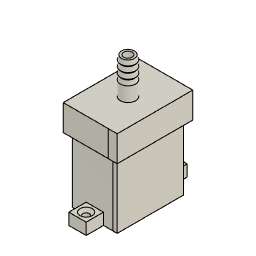
BMP280box v1 (Autodesk Fusion 360 design; units mm, degrees)
Autodesk Fusion 360 part; units mm, degrees
sketch "Sketch1" plane through (0, 0, 0) normal (0, 0, 1) x (1, 0, 0)
  line L0 (0, 0) -> (25, 0)
  line L1 (25, 0) -> (25, 40)
  line L2 (25, 40) -> (0, 40)
  line L3 (0, 40) -> (0, 0)
  line L4 (-3, 43) -> (-3, -3)
  line L5 (-3, -3) -> (28, -3)
  line L6 (28, -3) -> (28, 43)
  line L7 (28, 43) -> (-3, 43)
  line L8 (25, 40) -> (25, 43)
  line L9 (25, 0) -> (25, -3)
  line L10 (23.5, 24) -> (25, 24)
  line L11 (25, 24) -> (25, 16)
  line L12 (25, 16) -> (23.5, 16)
  line L13 (23.5, 16) -> (23.5, 24)
  line L14 (25, 35) -> (22, 35)
  line L15 (22, 35) -> (22, 32)
  line L16 (22, 32) -> (25, 32)
  line L17 (25, 32) -> (25, 35)
  line L18 (0, 20) -> (28, 20) construction
  line L19 (22, 8) -> (25, 8)
  line L20 (25, 8) -> (25, 5)
  line L21 (22, 5) -> (22, 8)
  line L22 (25, 5) -> (22, 5)
  line L23 (25, 4.8) -> (21.8, 4.8)
  line L24 (21.8, 4.8) -> (21.8, 8.2)
  line L25 (21.8, 8.2) -> (25, 8.2)
  line L26 (25, 35.2) -> (21.8, 35.2)
  line L27 (21.8, 35.2) -> (21.8, 31.8)
  line L28 (21.8, 31.8) -> (25, 31.8)
  dimension "d1" = 25
  dimension "d2" = 40
  dimension "d3" = 3
  dimension "d4" = 1.5
  dimension "d5" = 8
  dimension "d14" = 3
  dimension "d15" = 3
  dimension "d16" = 5
  dimension "d17" = -0.2
  dimension "d18" = 0.2
  constraint horizontal L0
  constraint vertical L1
  constraint horizontal L2
  constraint vertical L3
  constraint coincident L0.start L3.end
  constraint coincident L7 L8.end
  constraint perpendicular L7 L8
  constraint coincident L5 L9.end
  constraint perpendicular L5 L9
  constraint horizontal L10
  constraint vertical L11
  constraint horizontal L12
  constraint vertical L13
  constraint midpoint L1 L11
  constraint horizontal L14
  constraint vertical L15
  constraint horizontal L16
  constraint vertical L17
  constraint collinear L1 L17
  constraint midpoint L3 L18.start
  constraint midpoint L6 L18.end
  constraint symmetric L14.start L18 L20.end
  constraint symmetric L14.end L18 L21.start
  constraint symmetric L15.end L18 L19.start
  constraint symmetric L16.end L18 L19.end
  measures "d1" distance of L0.start L0.end
  measures "d2" distance of L0.start L2.end
  measures "d4" distance of L10.start L10.end
  measures "d5" distance of L10.start L12.end
  measures "d14" distance of L14.start L14.end
  measures "d15" distance of L14.start L16.end
  measures "d16" distance of L2 L14
  measures "d27" distance of L0.start
extrude "Extrude1" add sketch "Sketch1" against normal blind 20 contours L0 L1 L2 L3 L10 L12 L13 L23 L24 L25 L26 L27 L28 | L0 L2 L3 L4 L5 L7 L8 L9 makes body 1 in component "chambermainhalf"
extrude "Extrude2" add sketch "Sketch1" along normal blind 40 contours L0 L2 L3 L4 L5 L7 L8 L9 bodies 1 in component "chambermainhalf"
extrude "Extrude1'" add sketch "Sketch1" along normal up to surface (40 mm away) and the other way up to surface (20 mm away) separate body contours L1 L5 L6 L7 L8 L9 L11 L17 L20 makes body 2 in component "chambersealplate"
extrude "Extrude2'" add sketch "Sketch1" against normal up to surface (20 mm away) contours L1 L19 L20 L21 L22 | L1 L14 L15 L16 L17 bodies 2 in component "chambersealplate"
sketch "Sketch1 (2)" plane through (0, 0, 40) normal (0, 0, 1) x (-1, 0, 0) in component "ChamberLid"
  line L0 (-25, -40) -> (-25, -43)
  line L1 (-25, -43) -> (3, -43)
  line L2 (3, -43) -> (3, 3)
  line L3 (3, 3) -> (-25, 3)
  line L4 (-25, 3) -> (-25, 0)
  line L5 (-25, 0) -> (0, 0)
  line L6 (0, 0) -> (0, -40)
  line L7 (0, -40) -> (-25, -40)
  line L8 (-25, -43) -> (-25, 3)
  line L9 (-25, 3) -> (-28, 3)
  line L10 (-28, 3) -> (-28, -43)
  line L11 (-28, -43) -> (-25, -43)
  line L12 (3.2, 3.2) -> (-25, 3.2)
  line L13 (-25, 3.2) -> (-28.2, 3.2)
  line L14 (-28.2, 3.2) -> (-28.2, -43.2)
  line L15 (-28.2, -43.2) -> (-25, -43.2)
  line L16 (-25, -43.2) -> (3.2, -43.2)
  line L17 (3.2, -43.2) -> (3.2, 3.2)
  line L18 (6.2, 6.2) -> (-25, 6.2)
  line L19 (-25, 6.2) -> (-31.2, 6.2)
  line L20 (-31.2, 6.2) -> (-31.2, -46.2)
  line L21 (-31.2, -46.2) -> (-25, -46.2)
  line L22 (-25, -46.2) -> (6.2, -46.2)
  line L23 (6.2, -46.2) -> (6.2, 6.2)
  dimension "d19" = 0.2
  dimension "d20" = 3.2
extrude "Extrude1''" add sketch "Sketch1 (2)" against normal blind 15 separate body contours L18 L19 L20 L21 L22 L23 makes body 3 in component "ChamberLid"
sketch "Sketch2" plane through (0, 0, 40) normal (0, 0, 1) x (-1, 0, 0) in component "ChamberLid"
  line L0 (3.2, 3.2) -> (3.2, -43.2)
  line L1 (3.2, -43.2) -> (-25, -43.2)
  line L2 (-25, -43.2) -> (-28.2, -43.2)
  line L3 (-28.2, -43.2) -> (-28.2, 3.2)
  line L4 (-28.2, 3.2) -> (-25, 3.2)
  line L5 (-25, 3.2) -> (3.2, 3.2)
  line L6 (6.2, -46.2) -> (6.2, 6.2)
  line L7 (6.2, 6.2) -> (-25, 6.2)
  line L8 (-25, 6.2) -> (-31.2, 6.2)
  line L9 (-31.2, 6.2) -> (-31.2, -46.2)
  line L10 (-31.2, -46.2) -> (-25, -46.2)
  line L11 (-25, -46.2) -> (6.2, -46.2)
extrude "Extrude2''" add sketch "Sketch2" along normal blind 3 contours L0 L1 L2 L3 L4 L5 | L6 L7 L8 L9 L10 L11 bodies 3 in component "ChamberLid"
ref_plane "WorkPlane1" through (12.5, 20, 34) normal (-1, 0, 0) x (0, 1, 0) in component "ChamberLid"
sketch "Sketch3" plane through (12.5, 20, 34) normal (-1, 0, 0) x (0, 1, 0) in component "ChamberLid"
  line L0 (-26.2, -9) -> (26.2, -9)
  line L1 (0, -9) -> (0, -35) construction
  line L2 (5, -9) -> (5, -35) construction
  line L3 (4.5, -9) -> (3, -9)
  line L4 (3, -9) -> (3, -34)
  line L5 (3, -34) -> (4.5, -34)
  line L6 (4.5, -34) -> (4.5, -9)
  line L7 (4.5, -34) -> (5.3, -31)
  line L8 (5.3, -31) -> (4.5, -31)
  line L9 (5.3, -31) -> (4.5, -30.2)
  line L10 (4.5, -30) -> (5.3, -27)
  line L11 (5.3, -27) -> (4.5, -27)
  line L12 (5.3, -27) -> (4.5, -26.2)
  line L13 (4.5, -26) -> (5.3, -23)
  line L14 (5.3, -23) -> (4.5, -23)
  line L15 (5.3, -23) -> (4.5, -22.2)
  line L16 (4.5, -22) -> (5.3, -19)
  line L17 (5.3, -19) -> (4.5, -19)
  line L18 (5.3, -19) -> (4.5, -18.2)
  line L19 (5.3, -19) -> (5.3, -9)
  dimension "d25" = 5
  dimension "d26" = 1.5
  dimension "d27" = 25
  dimension "d28" = 0.5
  dimension "d29" = 3
  dimension "d30" = 0.8
  dimension "d31" = 45
  dimension "d34" = 0
  dimension "d35" = 4
  constraint midpoint L0 L1.start
  constraint perpendicular L0 L1
  constraint coincident L0 L2.start
  constraint perpendicular L0 L2
  constraint horizontal L3
  constraint vertical L4
  constraint horizontal L5
  constraint vertical L6
  constraint coincident L0 L3.start
  constraint coincident L6 L8.end
  constraint perpendicular L6 L8
  constraint coincident L6 L9.end
  constraint coincident L0 L19.end
  constraint perpendicular L0 L19
  measures "d25" distance of L1 L2
  measures "d26" distance of L4.end L5.end
  measures "d27" distance of L3.end L4.end
  measures "d28" distance of L2 L6
  measures "d29" vertical distance of L5.end L7.end
  measures "d30" distance of L7.end L8.end
  measures "d31" angle of L8 L9
revolve "Revolve1" add sketch "Sketch3" angle 360 about axis through (12.5, 20, 43) along (0, 0, 1) bodies 3 in component "ChamberLid"
extrude "Extrude3" cut 1 faces at (11.9171, 21.8898, 43) along direction (0, 0, -1) through all on bodies 3 bodies 3 in component "ChamberLid"
sketch "Sketch1 (3)" plane through (0, 0, -20) normal (0, 0, -1) x (1, 0, 0) in component "chambermainhalf"
  line L0 (25, -43) -> (25, -35.2)
  line L1 (25, -35.2) -> (21.8, -35.2)
  line L2 (21.8, -35.2) -> (21.8, -31.8)
  line L3 (21.8, -31.8) -> (25, -31.8)
  line L4 (25, -31.8) -> (25, -24)
  line L5 (25, -24) -> (23.5, -24)
  line L6 (23.5, -24) -> (23.5, -16)
  line L7 (23.5, -16) -> (25, -16)
  line L8 (25, -16) -> (25, -8.2)
  line L9 (25, -8.2) -> (21.8, -8.2)
  line L10 (21.8, -8.2) -> (21.8, -4.8)
  line L11 (21.8, -4.8) -> (25, -4.8)
  line L12 (25, -4.8) -> (25, 3)
  line L13 (25, 3) -> (-3, 3)
  line L14 (-3, 3) -> (-3, -43)
  line L15 (-3, -43) -> (25, -43)
  line L16 (6.5, 15) -> (18.5, 15)
  line L17 (18.5, 15) -> (18.5, 3)
  line L18 (18.5, 3) -> (6.5, 3)
  line L19 (6.5, 3) -> (6.5, 15)
  line L20 (28, 3) -> (25, 3) construction
  line L21 (25, 3) -> (25, -5) construction
  line L22 (25, -5) -> (22, -5) construction
  line L23 (22, -5) -> (22, -8) construction
  line L24 (22, -8) -> (25, -8) construction
  line L25 (25, -8) -> (25, -32) construction
  line L26 (25, -32) -> (22, -32) construction
  line L27 (22, -32) -> (22, -35) construction
  line L28 (22, -35) -> (25, -35) construction
  line L29 (25, -35) -> (25, -43) construction
  line L30 (25, -43) -> (28, -43) construction
  line L31 (28, -43) -> (28, 3) construction
  line L32 (28, 3) -> (-3, 3) construction
  line L33 (-3, -20) -> (23.5, -20) construction
  line L34 (6.5, -43) -> (6.5, -55)
  line L35 (18.5, -55) -> (18.5, -43)
  line L36 (18.5, -43) -> (6.5, -43)
  line L37 (6.5, -55) -> (18.5, -55)
  line L38 (12.5, 15) -> (12.5, 3) construction
  circle A0 centre (12.5, 9) radius 2.25
  circle A1 centre (12.5, -49) radius 2.25
  dimension "d40" = 12
  dimension "d41" = 12
  dimension "d44" = 4.5
  constraint horizontal L16
  constraint vertical L17
  constraint horizontal L18
  constraint vertical L19
  constraint coincident L20.start L31.end
  constraint coincident L13.end L14.start
  constraint midpoint L18 L32
  constraint midpoint L14 L33.start
  constraint midpoint L6 L33.end
  constraint symmetric L16.start L33 L34.end
  constraint symmetric L16.end L33 L35.start
  constraint symmetric L17.end L33 L35.end
  constraint symmetric L18.end L33 L34.start
  constraint midpoint L16 L38.start
  constraint midpoint L18 L38.end
  constraint midpoint L38 A0.centre
  constraint symmetric L33 A0 A1
  measures "d40" distance of L16.end L17.end
  measures "d41" distance of L16.start L16.end
  measures "d44" diameter of A0
extrude "Extrude3'" add sketch "Sketch1 (3)" against normal blind 8 contours L15 L34 L35 L36 L37 | L13 L16 L17 L18 L19 bodies 1 in component "chambermainhalf"
chamfer "Chamfer1" distance 2 angle 45 2 edges at (10.4023, -8.1864, -12) (10.4023, 49.8136, -12) on bodies 1 in component "chambermainhalf"
component "chambermainhalf" placed x (1, 0, 0) y (0, 1, 0) z (0, 0, 1) at (0, 0, 0)
component "chambersealplate" placed x (1, 0, 0) y (0, 1, 0) z (0, 0, 1) at (0, 0, 0)
component "ChamberLid" placed x (1, 0, 0) y (0, 1, 0) z (0, 0, 1) at (0, 0, 0)
